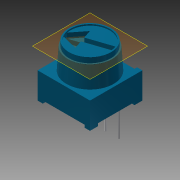
# Autodesk Inventor part: potentiometer
Saved by Autodesk Inventor 2015 (Build 190159000, 159)
## iProperties
Created: 2013-05-08
Part Number: potentiometer
Material: Generic
Document SubType Name: Modeling
Designer: Erika
Density: 1 g/cm^3
Appearance: Default
Author: Erika
Autodesk Inventor part; units mm, degrees
ref_plane "YZ Plane" through (0, 0, 0) normal (1, 0, 0) x (0, 1, 0)
ref_plane "XZ Plane" through (0, 0, 0) normal (0, 1, 0) x (-1, 0, 0)
ref_plane "XY Plane" through (0, 0, 0) normal (0, 0, 1) x (1, 0, 0)
sketch "Sketch1" plane through (0, 0, 0) normal (0, 0, 1) x (1, 0, 0)
  line L0 (-5, 5) -> (5, 5)
  line L1 (5, 5) -> (5, -5)
  line L2 (5, -5) -> (-5, -5)
  line L3 (-5, -5) -> (-5, 5)
  line L4 (-5, 5) -> (5, -5) construction
  line L5 (5, 5) -> (-5, -5) construction
  point P0 (0, 0)
  dimension "d0" = 10
  dimension "d2" = 10
  constraints: 12 end point, 2 midpoint, 2 parallel, 1 horizontal, 1 perpendicular
  measures "d0" distance of L0.end L1.end
  measures "d2" distance of L0.start L0.end
extrude "Extrusion1" add sketch "Sketch1" along normal blind 4.5
sketch "Sketch2" plane through (0, 0, 0) normal (0, 0, -1) x (-1, 0, 0)
  line L0 (-5, 5) -> (-4, 5)
  line L1 (-4, 5) -> (-4, 3.5)
  line L2 (-4, 3.5) -> (-5, 3.5)
  line L3 (-5, 3.5) -> (-5, 5)
  point P0 (0, 0)
  dimension "d5" = 1
  dimension "d6" = 1.5
  constraints: 8 end point, 2 parallel, 1 horizontal, 1 perpendicular
  measures "d5" distance of L0.start L0.end
  measures "d6" distance of L0.end L1.end
extrude "Extrusion2" add sketch "Sketch2" along normal blind 0.5
pattern_linear "Rectangular Pattern1" count 2 spacing 9 along (-1, 0, 0) count 2 spacing 8.5 along (0, -1, 0) of "Extrusion2"
sketch "Sketch3" plane through (-5, 5, 4.5) normal (0, 1, 0) x (1, 0, 0)
  line L0 (10, 0) -> (0, 0) projected
  line L1 (1, 4.5) -> (9, 4.5)
  line L2 (9, 4.5) -> (9, 0)
  line L3 (9, 0) -> (1, 0)
  line L4 (1, 0) -> (1, 4.5)
  point P0 (5, 4.5)
  constraints: 8 end point, 2 parallel, 1 horizontal, 1 perpendicular, 1 point on line
extrude "Extrusion3" cut sketch "Sketch3" against normal blind 0.5
sketch "Sketch4" plane through (0, 0, 0) normal (0, 0, -1) x (-1, 0, 0)
  line L0 (4, 4.5) -> (-4, 4.5) projected
  circle A0 centre (0, 3) radius 0.125
  circle A1 centre (2.5, 3) radius 0.125
  circle A2 centre (-2.5, 3) radius 0.125
  point P0 (0, 0)
  dimension "d17" = 2.5
  dimension "d19" = 2.5
  dimension "d20" = 0.25
  dimension "d21" = 1.5
  constraints: 3 centre point, 2 equal radius
  measures "d17" distance of A2.centre A0.centre
  measures "d19" distance of A1.centre A0.centre
  measures "d20" diameter of A1
  measures "d21" distance from line of L0 A1.centre
extrude "Extrusion4" add sketch "Sketch4" along normal blind 7
sketch "Sketch5" plane through (0, 0, 4.5) normal (0, 0, 1) x (1, 0, 0)
  circle A0 centre (0, 0) radius 4.5
  dimension "d25" = 9
  constraints: 1 centre point, 1 coincident
  measures "d25" diameter of A0
ref_plane "Work Plane1" through (0, 0, 8.5) normal (0, 0, 1) x (1, 0, 0)
sketch "Sketch6" plane through (0, 0, 8.5) normal (0, 0, 1) x (1, 0, 0)
  circle A0 centre (0, 0) radius 4.25
  dimension "d27" = 8.5
  constraints: 1 centre point, 1 coincident
  measures "d27" diameter of A0
loft "Loft1" add profiles "Sketch6", "Sketch5"
sketch "Sketch8" plane through (0, 0, 8.5) normal (0, 0, 1) x (1, 0, 0)
  circle A0 centre (0, 0) radius 4.25 projected
  circle A1 centre (0, 0) radius 4
  dimension "d34" = 8
  constraints: 1 centre point, 1 coincident
  measures "d34" diameter of A1
extrude "Extrusion5" add sketch "Sketch8" along normal blind 1 contours A1
sketch "Sketch9" plane through (0, 0, 9.5) normal (0, 0, 1) x (1, 0, 0)
  circle A0 centre (0, 0) radius 4 projected
  circle A1 centre (0, 0) radius 3.75
  dimension "d38" = 7.5
  constraints: 1 centre point, 1 coincident
  measures "d38" diameter of A1
extrude "Extrusion6" cut sketch "Sketch9" against normal blind 0.25 contours A1
sketch "Sketch10" plane through (0, 0, 9.25) normal (0, 0, 1) x (1, 0, 0)
  circle A0 centre (0, 0) radius 3.75 projected
  line L0 (3.7151, 0.7143) -> (-3.3982, -1.6628)
  line L1 (-3.3982, -1.6628) -> (-3.7151, -0.7143)
  line L2 (-3.7151, -0.7143) -> (3.3982, 1.6628)
  line L3 (3.3982, 1.6628) -> (3.7151, 0.7143)
  line L4 (3.7151, 0.7143) -> (-3.7151, -0.7143) construction
  line L5 (-3.3982, -1.6628) -> (3.3982, 1.6628) construction
  dimension "d42" = 1
  dimension "d44" = 7.5
  constraints: 12 end point, 2 midpoint, 2 parallel, 1 perpendicular
  measures "d42" distance between parallel lines of L0 L2
  measures "d44" distance between parallel lines of L3 L1
extrude "Extrusion7" cut sketch "Sketch10" against normal blind 2 contours L0 A0 L2 | A0 L3 L0 | L0 L1 A0 | A0 L2 L3 | L1 L2 A0
sketch "Sketch11" plane through (0, 0, 9.25) normal (0, 0, 1) x (1, 0, 0)
  line L0 (3.6834, 0.7037) -> (-3.3664, -1.6522) projected
  line L1 (-3.3664, -1.6522) -> (-0.3664, -2.446)
  line L2 (-0.3664, -2.446) -> (-0.9064, -0.8301)
  dimension "d49" = 3
  dimension "d51" = 56.7
  dimension "d53" = 1.6159
  constraints: 4 end point, 1 perpendicular, 1 point on line
  measures "d49" horizontal distance of L0.end L1.end
  measures "d51" angle of L2 L1
  measures "d53" vertical distance of L1.end L2.end
extrude "Extrusion8" cut sketch "Sketch11" against normal blind 1
sketch "Sketch13" plane through (0, 0, 9.25) normal (0, 0, 1) x (1, 0, 0)
  arc A0 (3.3664, 1.6522) -> (-3.6834, -0.7037) centre (0, 0) ccw projected
  line L0 (3.6834, 0.7037) -> (-3.3664, -1.6522)
  line L1 (-3.3664, -1.6522) -> (-0.3664, -2.446)
  line L2 (-0.3664, -2.446) -> (-0.9064, -0.8301)
  line L3 (0, 0) -> (-3.5718, -1.1936)
  line L4 (3.3664, 1.6522) -> (-3.6834, -0.7037)
  line L5 (-3.6834, -0.7037) -> (-1.7634, 1.7343)
  line L6 (-1.7634, 1.7343) -> (-1.2234, 0.1184)
  dimension "d55" = 3
  dimension "d56" = 56.7
  dimension "d57" = 1.6159
  constraints: 14 end point, 2 perpendicular, 2 point on line, 2 symmetric about line
  measures "d55" horizontal distance of L0.end L1.end
  measures "d56" angle of L2 L1
  measures "d57" vertical distance of L1.end L2.end
extrude "Extrusion9" cut sketch "Sketch13" against normal blind 1 contours L5 L6 L4
body "Solid1"
